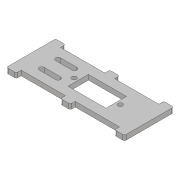
# Autodesk Inventor part: Side_Plate
Saved by Autodesk Inventor 2019 (Build 230136000, 136)
## iProperties
Created: 2021-06-25
Part Number: Side_Plate
Material: Generic
Document SubType Name: Modeling
Designer: Oudenas
Density: 1 g/cm^3
Appearance: Default
Mass: 4.25745 g
Surface Area: 40.2615 cm^2
Volume: 4.25745 cm^3
Sheet Metal Rule: Default
Author: Oudenas
Autodesk Inventor part; units mm, degrees
ref_plane "YZ Plane" through (0, 0, 0) normal (1, 0, 0) x (0, 1, 0)
ref_plane "XZ Plane" through (0, 0, 0) normal (0, 1, 0) x (-1, 0, 0)
ref_plane "XY Plane" through (0, 0, 0) normal (0, 0, 1) x (1, 0, 0)
sketch "Sketch1" plane through (0, 0, 0) normal (0, 1, 0) x (-1, 0, 0)
  line L0 (36, 15) -> (-36, 15)
  line L1 (-36, 15) -> (-36, -15)
  line L2 (-36, -15) -> (36, -15)
  line L3 (36, -15) -> (36, 15)
  line L4 (36, 15) -> (-36, -15) construction
  line L5 (-36, 15) -> (36, -15) construction
  point P0 (0, 0)
  dimension "d0" = 72
  dimension "d1" = 30
  constraints: 12 end point, 2 midpoint, 2 parallel, 1 horizontal, 1 perpendicular
  measures "d0" distance of L2.end L1.end
  measures "d1" distance of L1.end L0.end
extrude "Extrusion1" add sketch "Sketch1" along normal blind 3
sketch "Sketch2" plane through (0, 3, 0) normal (0, 1, 0) x (1, 0, 0)
  line L0 (-7.2, 6.25) -> (16, 6.25)
  line L1 (16, 6.25) -> (16, -6.25)
  line L2 (16, -6.25) -> (-7.2, -6.25)
  line L3 (-7.2, -6.25) -> (-7.2, 6.25)
  line L4 (-7.2, 6.25) -> (16, -6.25) construction
  line L5 (16, 6.25) -> (-7.2, -6.25) construction
  line L6 (-36, 15) -> (-36, -15) projected
  line L7 (36, -15) -> (36, 15) projected
  line L8 (36, 15) -> (-36, 15) projected
  line L9 (-36, -15) -> (36, -15) projected
  point P0 (0, 0)
  point P1 (4.4, 0)
  point P2 (4.4, 0)
  dimension "d5" = 20
  dimension "d33" = 12.5
  dimension "d34" = 23.2
  constraints: 12 end point, 3 midpoint, 2 parallel, 1 horizontal, 1 horizontal alignment, 1 perpendicular
  measures "d5" distance between parallel lines of L7 L1
  measures "d33" distance between parallel lines of L2 L0
  measures "d34" distance between parallel lines of L1 L3
extrude "Extrusion2" cut sketch "Sketch2" against normal blind 3 contours L0 L1 L2 L3
sketch "Sketch3" plane through (0, 3, 0) normal (0, 1, 0) x (1, 0, 0)
  line L0 (-30, 18) -> (30, 18)
  line L1 (30, 18) -> (30, 12)
  line L2 (30, 12) -> (-30, 12)
  line L3 (-30, 12) -> (-30, 18)
  line L4 (36, 15) -> (-36, 15) projected
  line L5 (-30, 18) -> (30, 12) construction
  line L6 (30, 18) -> (-30, 12) construction
  line L7 (-30, -12) -> (30, -12)
  line L8 (30, -12) -> (30, -18)
  line L9 (30, -18) -> (-30, -18)
  line L10 (-30, -18) -> (-30, -12)
  line L11 (-36, -15) -> (36, -15) projected
  line L12 (-30, -12) -> (30, -18) construction
  line L13 (30, -12) -> (-30, -18) construction
  point P0 (0, 0)
  point P1 (0, 15)
  point P2 (0, -15)
  dimension "d10" = 60
  dimension "d11" = 6
  dimension "d12" = 60
  dimension "d13" = 6
  constraints: 24 end point, 6 midpoint, 4 parallel, 2 horizontal, 2 perpendicular
  measures "d10" distance of L1.end L2.end
  measures "d11" distance of L0.end L1.end
  measures "d12" distance of L8.end L9.end
  measures "d13" distance of L7.end L8.end
extrude "Extrusion3" cut sketch "Sketch3" against normal blind 3
sketch "Sketch4" plane through (0, 0, 0) normal (0, -1, 0) x (1, 0, 0)
  circle A0 centre (18.5, 0) radius 1.45
  circle A1 centre (-9.7, 0) radius 1.45
  line L0 (-7.2, -6.25) -> (-7.2, 6.25) projected
  line L1 (16, 6.25) -> (16, -6.25) projected
  line L2 (-7.2, 6.25) -> (16, 6.25) projected
  line L3 (16, -6.25) -> (-7.2, -6.25) projected
  line L4 (-30, -12) -> (30, -12) projected
  line L5 (30, 12) -> (-30, 12) projected
  point P0 (0, 0)
  dimension "d16" = 2.9
  dimension "d18" = 2.9
  dimension "d20" = 2.5
  dimension "d21" = 2.5
  constraints: 2 centre point, 2 horizontal alignment
  measures "d16" diameter of A0
  measures "d18" diameter of A1
  measures "d20" distance from line of A1.centre L0
  measures "d21" distance from line of L1 A0.centre
extrude "Extrusion4" cut sketch "Sketch4" against normal blind 3 contours A0 | A1
sketch "Sketch5" plane through (0, 0, 0) normal (0, -1, 0) x (1, 0, 0)
  line L0 (3, 15) -> (-3, 15)
  line L1 (-3, 15) -> (-3, 11)
  line L2 (-3, -15) -> (3, -15)
  line L3 (3, -15) -> (3, -11)
  line L4 (3, -11) -> (-3, -11)
  line L5 (3, 11) -> (-3, 11)
  line L6 (3, 11) -> (3, 15)
  line L7 (-3, -11) -> (-3, -15)
  line L8 (30, 12) -> (-30, 12) projected
  line L9 (-30, -12) -> (30, -12) projected
  point P0 (0, 0)
  dimension "d26" = 6
  dimension "d35" = 6
  dimension "d36" = 4
  dimension "d37" = 3
  dimension "d38" = 3
  dimension "d39" = 4
  constraints: 16 end point, 5 parallel, 2 perpendicular, 1 point on line
  measures "d26" distance of L2.end L2.start
  measures "d35" distance between parallel lines of L1 L6
  measures "d36" distance between parallel lines of L5 L0
  measures "d37" distance between parallel lines of L8 L0
  measures "d38" distance between parallel lines of L9 L2
  measures "d39" distance between parallel lines of L2 L4
extrude "Extrusion5" add sketch "Sketch5" against normal blind 3
fillet "Fillet1" radius 1 12 edges at (-30, 1.5, 15) (-36, 1.5, 15) (-3, 1.5, 15) (3, 1.5, 15) (30, 1.5, 15) (36, 1.5, 15) (36, 1.5, -15) (30, 1.5, -15) (-3, 1.5, -15) (3, 1.5, -15) (-30, 1.5, -15) (-36, 1.5, -15)
sketch "Sketch6" plane through (0, 0, 0) normal (0, -1, 0) x (1, 0, 0)
  line L0 (-36, -14) -> (-36, 14) projected
  line L1 (-30, -12) -> (-3, -12) projected
  line L2 (-14.5, -5) -> (-24.5, -5) construction
  line L3 (-14.5, -3.5) -> (-24.5, -3.5)
  line L4 (-24.5, -6.5) -> (-14.5, -6.5)
  arc A0 (-14.5, -6.5) -> (-14.5, -3.5) centre (-14.5, -5) ccw
  arc A1 (-24.5, -3.5) -> (-24.5, -6.5) centre (-24.5, -5) ccw
  line L5 (-14.5, 5) -> (-24.5, 5) construction
  line L6 (-14.5, 6.5) -> (-24.5, 6.5)
  line L7 (-24.5, 3.5) -> (-14.5, 3.5)
  arc A2 (-14.5, 3.5) -> (-14.5, 6.5) centre (-14.5, 5) ccw
  arc A3 (-24.5, 6.5) -> (-24.5, 3.5) centre (-24.5, 5) ccw
  line L8 (-3, 12) -> (-30, 12) projected
  point P0 (0, 0)
  point P1 (-19.5, 5)
  point P2 (-19.5, -5)
  dimension "d47" = 3
  dimension "d48" = 5
  dimension "d49" = 3
  dimension "d50" = 7
  dimension "d51" = 5
  dimension "d52" = 16.5
  constraints: 16 end point, 8 point on circle, 8 tangent, 4 centre point, 2 midpoint, 2 parallel, 1 horizontal, 1 vertical alignment
  measures "d47" diameter of A1
  measures "d48" distance of point (-19.5, 5) L5.end
  measures "d49" diameter of A3
  measures "d50" distance from line of L8 point (-19.5, 5)
  measures "d51" distance of point (-19.5, -5) L2.end
  measures "d52" distance from line of L0 point (-19.5, 5)
extrude "Extrusion6" cut sketch "Sketch6" against normal blind 10
sketch "Sketch8" plane through (0, 0, 0) normal (0, -1, 0) x (1, 0, 0)
  line L0 (-26.5433, -8.3077) -> (-29.9566, -8.3077) construction
  line L1 (-29.9566, -8.3077) -> (-29.9566, -4.3077) construction
  line L2 (-29.9566, -4.3077) -> (-26.5433, -4.3077) construction
  line L3 (-26.5433, -4.3077) -> (-26.5433, -8.3077) construction
  line L4 (-29.371, 1.4831) -> (-29.371, -2.5169) construction
  line L5 (-29.371, -2.5169) -> (-32.7843, -2.5169) construction
  line L6 (-32.7843, -2.5169) -> (-32.7843, 1.4831) construction
  line L7 (-32.7843, 1.4831) -> (-29.371, 1.4831) construction
  line L8 (-31.6431, 4.0727) -> (-31.6431, 8.0727) construction
  line L9 (-31.6431, 8.0727) -> (-28.2298, 8.0727) construction
  line L10 (-28.2298, 8.0727) -> (-28.2298, 4.0727) construction
  line L11 (-28.2298, 4.0727) -> (-31.6431, 4.0727) construction
  spline S0 degree 2 poles (-31.6212, -4.4316) (-31.6212, -4.3978) (-31.5837, -4.3528) (-31.4447, -4.319) (-31.178, -4.3077) (-30.9452, -4.3077) knots 0 0 0 1 2 3 4 4 4
  spline S1 degree 2 poles (-30.9452, -4.3077) (-30.7536, -4.3077) (-30.5208, -4.319) (-30.3893, -4.3528) (-30.333, -4.4053) (-30.3142, -4.4429) knots 0 0 0 1 2 3 4 4 4
  line L12 (-30.3142, -4.4429) -> (-29.7809, -5.333)
  spline S2 degree 2 poles (-29.7809, -5.333) (-29.6832, -5.4833) (-29.4992, -5.7161) (-29.2738, -5.8739) (-28.9771, -5.9528) (-28.7856, -5.9528) knots 0 0 0 1 2 3 4 4 4
  line L13 (-28.7856, -5.9528) -> (-28.4062, -5.9528)
  line L14 (-28.4062, -5.9528) -> (-28.4062, -4.4392)
  spline S3 degree 2 poles (-28.4062, -4.4392) (-28.4062, -4.4053) (-28.3461, -4.3565) (-28.2072, -4.3265) (-27.978, -4.3077) (-27.7978, -4.3077) knots 0 0 0 1 2 3 4 4 4
  spline S4 degree 2 poles (-27.7978, -4.3077) (-27.6212, -4.3077) (-27.3884, -4.3265) (-27.2494, -4.3565) (-27.1931, -4.4053) (-27.1931, -4.4392) knots 0 0 0 1 2 3 4 4 4
  line L15 (-27.1931, -4.4392) -> (-27.1931, -8.0523)
  spline S5 degree 2 poles (-27.1931, -8.0523) (-27.1931, -8.1875) (-27.3996, -8.3077) (-27.5536, -8.3077) knots 0 0 0 1 2 2 2
  line L16 (-27.5536, -8.3077) -> (-29.0973, -8.3077)
  spline S6 degree 2 poles (-29.0973, -8.3077) (-29.3339, -8.3077) (-29.6381, -8.2964) (-29.7621, -8.2852) knots 0 0 0 1 2 2 2
  spline S7 degree 2 poles (-29.7621, -8.2852) (-30.1226, -8.2514) (-30.6973, -8.0861) (-31.0992, -7.8194) (-31.3095, -7.4514) (-31.3095, -7.2147) knots 0 0 0 1 2 3 4 4 4
  spline S8 degree 2 poles (-31.3095, -7.2147) (-31.3095, -7.0157) (-31.1593, -6.6852) (-30.8625, -6.4298) (-30.4306, -6.2382) (-30.1527, -6.1781) knots 0 0 0 1 2 3 4 4 4
  spline S9 degree 2 poles (-30.1527, -6.1781) (-30.2879, -6.1368) (-30.5208, -6.0129) (-30.7311, -5.8363) (-30.9151, -5.611) (-31.0015, -5.472) knots 0 0 0 1 2 3 4 4 4
  line L17 (-31.0015, -5.472) -> (-31.5048, -4.687)
  spline S10 degree 2 poles (-31.5048, -4.687) (-31.5724, -4.5706) (-31.6212, -4.4617) (-31.6212, -4.4316) knots 0 0 0 1 2 2 2
  spline S11 degree 2 poles (-30.055, -7.1321) (-30.055, -7.3312) (-29.7884, -7.6016) (-29.4841, -7.6579) knots 0 0 0 1 2 2 2
  spline S12 degree 2 poles (-29.4841, -7.6579) (-29.394, -7.673) (-29.1574, -7.6917) (-28.9508, -7.6917) knots 0 0 0 1 2 2 2
  line L18 (-28.9508, -7.6917) -> (-28.4062, -7.6917)
  line L19 (-28.4062, -7.6917) -> (-28.4062, -6.5612)
  line L20 (-28.4062, -6.5612) -> (-29.0222, -6.5612)
  spline S13 degree 2 poles (-29.0222, -6.5612) (-29.2813, -6.5612) (-29.6682, -6.6438) (-29.9273, -6.7941) (-30.055, -7.0044) (-30.055, -7.1321) knots 0 0 0 1 2 3 4 4 4
  line L21 (-29.7593, -2.5169) -> (-34.7608, -0.0162)
  line L22 (-34.7608, -0.0162) -> (-29.7593, 2.4754)
  line L23 (-29.7593, 2.4754) -> (-29.7593, 1.574)
  line L24 (-29.7593, 1.574) -> (-33.069, -0.0162)
  line L25 (-33.069, -0.0162) -> (-29.7593, -1.6109)
  line L26 (-29.7593, -1.6109) -> (-29.7593, -2.5169)
  spline S14 degree 2 poles (-27.7145, 4.4107) (-27.7145, 4.3206) (-27.737, 4.1929) (-27.7858, 4.1102) (-27.8534, 4.0727) (-27.8985, 4.0727) knots 0 0 0 1 2 3 4 4 4
  line L27 (-27.8985, 4.0727) -> (-30.6328, 4.0727)
  spline S15 degree 2 poles (-30.6328, 4.0727) (-30.7868, 4.0727) (-30.9933, 4.1929) (-30.9933, 4.3281) knots 0 0 0 1 2 2 2
  line L28 (-30.9933, 4.3281) -> (-30.9933, 7.945)
  spline S16 degree 2 poles (-30.9933, 7.945) (-30.9933, 7.975) (-30.9332, 8.0238) (-30.7943, 8.0539) (-30.5614, 8.0727) (-30.3849, 8.0727) knots 0 0 0 1 2 3 4 4 4
  spline S17 degree 2 poles (-30.3849, 8.0727) (-30.2046, 8.0727) (-29.9755, 8.0539) (-29.8365, 8.0238) (-29.7764, 7.975) (-29.7764, 7.945) knots 0 0 0 1 2 3 4 4 4
  line L29 (-29.7764, 7.945) -> (-29.7764, 4.7412)
  line L30 (-29.7764, 4.7412) -> (-27.8985, 4.7412)
  spline S18 degree 2 poles (-27.8985, 4.7412) (-27.8534, 4.7412) (-27.7858, 4.7074) (-27.737, 4.6285) (-27.7145, 4.5046) (-27.7145, 4.4107) knots 0 0 0 1 2 3 4 4 4
  point P0 (0, 0)
  constraints: 6 other
extrude "Extrusion8" cut sketch "Sketch8" against normal blind 0.6
fillet "Fillet2" radius 0.2 17 edges at (-30.3142, 0.3, -4.4429) (-28.4062, 0.3, -4.4392) (-31.0015, 0.3, -5.472) (-28.4062, 0.3, -5.9528) (-30.1527, 0.3, -6.1781) (-27.7978, 0.3, -4.3077) (-29.7809, 0.3, -5.333) (-28.7856, 0.3, -5.9528) (-28.4062, 0.3, -7.6917) (-33.069, 0.3, -0.0162) (-29.7593, 0.3, 1.574) (-29.7593, 0.3, 2.4754) (-29.7593, 0.3, -1.6109) (-29.7593, 0.3, -2.5169) (-34.7608, 0.3, -0.0162) (-28.4062, 0.3, -6.5612) (-29.7764, 0.3, 4.7412)
equation "\"d16\" = d18"
equation "\"d20\" = d21"
equation "\"d51\" = d48"
equation "\"BendRadius\" = Thickness"
equation "\"BendReliefWidth\" = Thickness"
equation "\"BendReliefDepth\" = 0.5 * Thickness"
equation "\"CornerReliefSize\" = 4 * Thickness"
equation "\"MinimumRemnant\" = 2 * Thickness"
equation "\"TransitionRadius\" = BendRadius"
equation "\"JacobiRadiusSize\" = Thickness"
equation "\"GapSize\" = Thickness"
equation "\"Thickness\" = 0.5"
body "Solid1"
